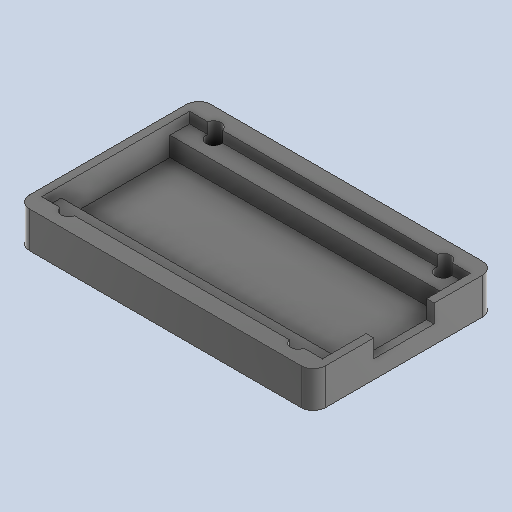
# Autodesk Inventor part: Voltmeter_lower_cover
Saved by Autodesk Inventor 2022.4 (Build 264492000, 492)
## iProperties
Created: 2021-10-13
Part Number: Voltmeter_lower_cover
Material: アセタール樹脂、黒
Document SubType Name: Modeling
Designer: Masato Kubotera
Density: 1.425 g/cm^3
Appearance: 滑らか - 黒
Description: PLA
Mass: 5.61048 g
Surface Area: 45.7612 cm^2
Volume: 3.93718 cm^3
Author: Masato Kubotera
Autodesk Inventor part; units mm, degrees
ref_plane "YZ Plane" through (0, 0, 0) normal (1, 0, 0) x (0, 1, 0)
ref_plane "XZ Plane" through (0, 0, 0) normal (0, 1, 0) x (-1, 0, 0)
ref_plane "XY Plane" through (0, 0, 0) normal (0, 0, 1) x (1, 0, 0)
derived "Voltmeter_basis.ipt"
sketch "スケッチ1" plane through (0, 0, 0) normal (0, 0, 1) x (1, 0, 0)
  line L0 (23, 12) -> (23, -12)
  line L1 (23, 12) -> (-23, -12) construction
  circle A0 centre (-19, 12) radius 3 construction
  line L2 (-23, 0) -> (23, 0) construction
  line L3 (0, 12) -> (0, -12) construction
  line L4 (-23, 12) -> (23, -12) construction
  line L5 (-23, 12) -> (-20.6, 12)
  arc A1 (-20.6, 12) -> (-17.4, 12) centre (-19, 12) ccw
  arc A2 (-17.4, -12) -> (-20.6, -12) centre (-19, -12) ccw
  line L6 (-23, -12) -> (-20.6, -12)
  arc A3 (17.4, 12) -> (20.6, 12) centre (19, 12) ccw
  line L7 (23, 12) -> (20.6, 12)
  line L8 (23, -12) -> (20.6, -12)
  arc A4 (20.6, -12) -> (17.4, -12) centre (19, -12) ccw
  line L9 (-17.4, 12) -> (17.4, 12)
  line L10 (17.4, -12) -> (-17.4, -12)
  line L11 (-23, 12) -> (-23, -12)
  line L12 (-24.5, 15) -> (24.5, 15)
  line L13 (24.5, 15) -> (24.5, -15)
  line L14 (24.5, -15) -> (-24.5, -15)
  line L15 (-24.5, -15) -> (-24.5, 15)
  line L16 (-24.5, 15) -> (24.5, -15) construction
  line L17 (24.5, 15) -> (-24.5, -15) construction
  line L18 (-23.25, 12.25) -> (23.25, 12.25)
  line L19 (23.25, 12.25) -> (23.25, -12.25)
  line L20 (23.25, -12.25) -> (-23.25, -12.25)
  line L21 (-23.25, -12.25) -> (-23.25, 12.25)
  line L22 (-23.25, 12.25) -> (23.25, -12.25) construction
  line L23 (23.25, 12.25) -> (-23.25, -12.25) construction
  circle A5 centre (19, 12) radius 3 construction
  circle A6 centre (-19, -12) radius 3 construction
  circle A7 centre (19, -12) radius 3 construction
  circle A8 centre (-19, 12) radius 1.25
  circle A9 centre (19, 12) radius 1.25
  circle A10 centre (-19, -12) radius 1.25
  circle A11 centre (19, -12) radius 1.25
  line L24 (-23.25, 9) -> (23.25, 9)
  line L25 (-23.25, -9) -> (23.25, -9)
  line L26 (24.5, 5) -> (23.25, 5)
  line L27 (24.5, -5) -> (23.25, -5)
  point P0 (0, 0)
  point P1 (0, 0)
  point P2 (0, 0)
  point P3 (20.2247, -12.25)
  point P4 (17.7753, -12.25)
  point P5 (-17.7753, -12.25)
  point P6 (-20.2247, -12.25)
  point P7 (-20.2247, 12.25)
  point P8 (-17.7753, 12.25)
  point P9 (17.7753, 12.25)
  point P10 (20.2247, 12.25)
  dimension "d3" = 2.5
  dimension "d4" = 2.5
  dimension "d5" = 2.5
  dimension "d6" = 2.5
  dimension "d8" = 18
  dimension "d9" = 10
  measures "d3" diameter of A8
  measures "d4" diameter of A9
  measures "d5" diameter of A10
  measures "d6" diameter of A11
  measures "d8" distance of L25.end L24.end
  measures "d9" distance of L27.start L26.start
extrude "押し出し1" add sketch "スケッチ1" along normal blind 6 contours L19 L18 A9 A8 L21 L20 A10 A11 L27 L13 L14 L15 L12 L26
extrude "押し出し2" add sketch "スケッチ1" along normal blind 4.2 contours L7 A3 L9 A1 L5 L11 L24 L21 L18 A8 A9 L19 L0 | L0 L24 L11 L5 A1 L9 A3 L7 | L25 L19 L20 A11 A10 L21 L11 L6 A2 L10 A4 L8 L0 | L0 L8 A4 L10 A2 L6 L11 L25
extrude "押し出し3" add sketch "スケッチ1" along normal blind 1 contours L24 L19 L25 L0 | L0 L25 L11 L24 | L11 L25 L21 L24
extrude "押し出し4" add sketch "スケッチ1" along normal blind 3 contours L26 L13 L27 L19
fillet "フィレット1" radius 2 4 edges at (-24.5, -15, 3) (-24.5, 15, 3) (24.5, 15, 3) (24.5, -15, 3)
equation "\"d4\" = d3"
equation "\"d5\" = d3"
equation "\"d6\" = d3"
